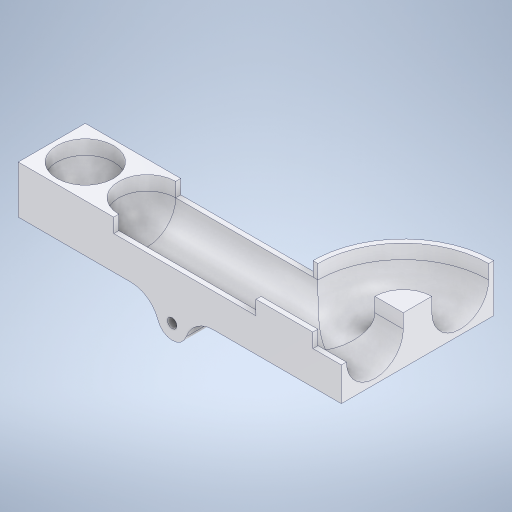
# Autodesk Inventor part: Trilho 5 min
Saved by Autodesk Inventor 2024 (Build 280153000, 153)
## iProperties
Created: 2023-05-15
Part Number: Trilho 5 min
Material: Plástico PET
Document SubType Name: Modeling
Designer: jpjoa
Density: 1.541 g/cm^3
Appearance: PTFE
Mass: 26.187 g
Surface Area: 115.473 cm^2
Volume: 16.9935 cm^3
Author: jpjoa
Autodesk Inventor part; units mm, degrees
ref_plane "YZ Plane" through (0, 0, 0) normal (1, 0, 0) x (0, 1, 0)
ref_plane "XZ Plane" through (0, 0, 0) normal (0, 1, 0) x (-1, 0, 0)
ref_plane "XY Plane" through (0, 0, 0) normal (0, 0, 1) x (1, 0, 0)
sketch "Esboço1" plane through (0, 0, 0) normal (0, 1, 0) x (-1, 0, 0)
  arc A0 (-102.2, -28.6) -> (-93.2, -19.6) centre (-102.2, -19.6) ccw
  arc A1 (-102.2, -46.6) -> (-75.2, -19.6) centre (-102.2, -19.6) ccw
  line L0 (-75.2, -19.6) -> (-30.2, -19.6)
  line L1 (-93.2, -19.6) -> (-102.2, -19.6)
  line L2 (-102.2, -19.6) -> (-102.2, -1.6)
  line L3 (-102.2, -1.6) -> (-93.2, -1.6)
  line L4 (-93.2, -1.6) -> (-75.2, -1.6)
  line L5 (-75.2, -1.6) -> (-30.2, -1.6)
  arc A2 (-30.2, -19.6) -> (-30.2, -1.6) centre (-30.2, -10.6) ccw
  line L6 (-102.2, -28.6) -> (-102.2, -46.6)
  arc A3 (-102.2, -48.2) -> (-73.6448, -21.2) centre (-102.2, -19.6) ccw
  arc A4 (-102.2, -27) -> (-94.975, -21.2) centre (-102.2, -19.6) ccw
  line L7 (-94.975, -21.2) -> (-102.2, -21.2)
  line L8 (-102.2, 0) -> (-93.2, 0)
  line L9 (-93.2, 0) -> (-75.2, 0)
  line L10 (-75.2, 0) -> (0, 0)
  line L11 (0, -21.2) -> (-73.6448, -21.2)
  line L12 (-73.6448, -21.2) -> (-73.6448, -19.6)
  line L13 (-102.2, -46.6) -> (-102.2, -48.2)
  line L14 (-102.2, -28.6) -> (-102.2, -27)
  line L15 (-102.2, -21.2) -> (-102.2, -19.6)
  line L16 (-102.2, -1.6) -> (-102.2, 0)
  line L17 (-94.975, -21.2) -> (-94.975, -19.6)
  line L18 (-93.2, -1.6) -> (-93.2, 0)
  line L19 (-75.2, -1.6) -> (-75.2, 0)
  line L20 (0, -21.2) -> (0, 0)
  circle A5 centre (-10.6, -10.6) radius 9
  line L21 (-30.2, -21.2) -> (-30.2, -19.6)
  line L22 (-30.2, -1.6) -> (-30.2, 0)
  line L23 (-102.2, -21.2) -> (-102.2, -27)
  point P0 (-21.2, -10.6)
  point P1 (-73.6448, -21.2)
  point P2 (-30.2, -1.6)
  point P3 (-30.2, -19.6)
  dimension "d20" = 18
  dimension "d21" = 18
  dimension "d22" = 54
  dimension "d23" = 1.6
  dimension "d30" = 1.6
  dimension "d31" = 1.6
  dimension "d32" = 1.6
  dimension "d33" = 9
  dimension "d35" = 18
  dimension "d38" = 1.6
  dimension "d44" = 1.6
  dimension "d45" = 1.6
  constraints: 48 end point, 15 point on circle, 12 coincident, 12 point on line, 11 vertical, 11 vertical alignment, 7 horizontal alignment, 6 centre point, 2 horizontal, 2 tangent, 1 line through centre, 1 perpendicular, 1 other
  measures "d20" radial gap between concentric circles of A0 A1
  measures "d21" diameter of A2
  measures "d22" horizontal distance of point (-21.2, -10.6) L0.start
  measures "d23" radial gap between concentric circles of A1 A3
  measures "d30" distance between parallel lines of L11 L0
  measures "d31" radial gap between concentric circles of A0 A4
  measures "d32" distance between parallel lines of L1 L7
  measures "d33" distance of L1.start L1.end
  measures "d35" diameter of A5
  measures "d38" distance edge to line of A5 L20
  measures "d45" distance between parallel lines of L10 L5
extrude "Margem externa" add sketch "Esboço1" against normal blind 1.6 contours L14 A4 L17 L1 A0 | A0 L1 L2 L3 L4 L5 A2 L0 A1 L6 | A1 L0 L12 A3 L13 | L23 L7 A4 | L17 L7 L15 L1 | L0 L21 L11 L12 | L16 L8 L18 L3 | A2 L22 L10 L20 L11 L21 | L18 L9 L19 L4 | L5 L19 L10 L22 | A5
extrude "Proteção alta" add sketch "Esboço1" along normal blind 13.5 contours L14 A4 L17 L1 A0 | A1 L0 L12 A3 L13 | L23 L7 A4 | L17 L7 L15 L1 | A2 L22 L10 L20 L11 L21 | L18 L9 L19 L4
extrude "Proteção baixa" add sketch "Esboço1" along normal blind 9 contours L14 A4 L17 L1 A0 | A1 L0 L12 A3 L13 | L17 L7 L15 L1 | L0 L21 L11 L12 | L16 L8 L18 L3 | A2 L22 L10 L20 L11 L21 | L18 L9 L19 L4 | L5 L19 L10 L22
fillet "Arredondamento3" radius 9 7 edges at (19.6, 0, -10.6) (66.2, 0, -1.6) (52.7, 0, -19.6) (21.2, 0, -10.6) (83.1081, 0, -38.6919) (97.7, 0, -19.6) (95.836, 0, -25.964)
sketch "Esboço2" plane through (0, -1.6, 0) normal (0, -1, 0) x (1, 0, 0)
  line L0 (56.187, 0) -> (41.187, 0)
  line L1 (41.187, 0) -> (41.187, -10.6)
  line L2 (41.187, -10.6) -> (56.187, -10.6)
  line L3 (56.187, -10.6) -> (56.187, 0)
  line L4 (0, 0) -> (0, -21.2) projected
  point P0 (48.687, -10.6)
  point P1 (0, -10.6)
  point P2 (48.687, 0)
  dimension "d47" = 48.687
  dimension "d48" = 15
  constraints: 8 end point, 3 midpoint, 3 perpendicular, 2 horizontal alignment, 1 horizontal
  measures "d47" distance from line of L4 point (48.687, -10.6)
  measures "d48" distance between parallel lines of L3 L1
extrude "Extrusão5" add sketch "Esboço2" along normal blind 9.4
sketch "Esboço3" plane through (56.187, -1.6, -10.6) normal (0, 0, -1) x (-1, 0, 0)
  circle A0 centre (7.5, -4.7) radius 1.5
  line L0 (15, -9.4) -> (0, -9.4) projected
  line L1 (15, 0) -> (15, -9.4) projected
  line L2 (56.187, 0) -> (-17.4578, 0) projected
  line L3 (12.2, 0) -> (15, 0)
  line L4 (15, 0) -> (15, -9.4)
  line L5 (15.1598, -9.4) -> (0, -9.4)
  line L6 (0, -9.4) -> (0, 0)
  line L7 (0, 0) -> (2.8, 0)
  circle A1 centre (7.5, -4.7) radius 4.7
  line L8 (12.2, 0) -> (12.2, -4.7)
  line L9 (2.8, 0) -> (2.8, -4.7)
  point P0 (56.187, 1.6)
  point P1 (7.5, -9.4)
  point P2 (15, -4.7)
  point P3 (9, -4.7)
  point P4 (6, -4.7)
  point P5 (7.5, -9.4)
  dimension "d51" = 3
  dimension "d54" = 3.2
  constraints: 14 end point, 4 perpendicular, 4 point on circle, 3 point on line, 2 centre point, 2 midpoint, 2 tangent, 2 vertical, 1 collinear, 1 horizontal alignment, 1 vertical alignment
  measures "d51" diameter of A0
  measures "d54" radial gap between concentric circles of A0 A1
extrude "Extrusão6" cut sketch "Esboço3" against normal through all contours A0 | L0 A1 L8 L2 L1 | L0 L6 L2 L9 A1
fillet "Arredondamento4" radius 9 2 edges at (53.387, -1.6, -5.3) (43.987, -1.6, -5.3)
equation "\"d20\" = Esfera"
equation "\"d21\" = Esfera"
equation "\"d22\" = 3 * Esfera"
equation "\"d23\" = Margem"
equation "\"d30\" = Margem"
equation "\"d31\" = Margem"
equation "\"d28\" = Margem"
equation "\"d24\" = 0.75 * Esfera"
equation "\"Esfera\" = 18"
equation "\"Margem\" = 1.6"
equation "\"Furo\" = 3"
